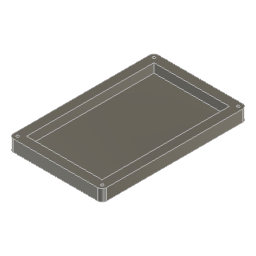
Veekos-bottom (Autodesk Fusion 360 design; units mm, degrees)
part number: 2026-09-15-13-32-07-212
Autodesk Fusion 360 part; units mm, degrees
sketch "Sketch1" plane through (0, 0, 0) normal (0, 0, 1) x (1, 0, 0)
  line L0 (-51.3011, 107.6317) -> (32.8009, 107.6317)
  line L1 (32.8009, 107.6317) -> (32.8009, -34.1263)
  line L2 (32.8009, -34.1263) -> (-51.3011, -34.1263)
  line L3 (-51.3011, -34.1263) -> (-51.3011, 107.6317)
  line L4 (-61.3011, 117.6317) -> (42.8009, 117.6317)
  line L5 (42.8009, 117.6317) -> (42.8009, -44.1263)
  line L6 (42.8009, -44.1263) -> (-61.3011, -44.1263)
  line L7 (-61.3011, -44.1263) -> (-61.3011, 117.6317)
  circle A0 centre (37.8009, 112.6317) radius 1.45
  circle A1 centre (37.8009, -39.1263) radius 1.45
  circle A2 centre (-56.3011, -39.1263) radius 1.45
  circle A3 centre (-56.3011, 112.6317) radius 1.45
  dimension "d1" = 84.102
  dimension "d2" = 141.758
  dimension "d3" = 104.102
  dimension "d4" = 161.758
  dimension "d5" = 10
  dimension "d6" = 10
  dimension "d7" = 2.9
  dimension "d8" = 5
  dimension "d9" = 5
  dimension "d10" = 2.9
  dimension "d11" = 5
  dimension "d12" = 5
  dimension "d13" = 2.9
  dimension "d14" = 5
  dimension "d15" = 5
  dimension "d16" = 2.9
  dimension "d17" = 5
  dimension "d18" = 5
  constraint horizontal L0
  constraint vertical L1
  constraint horizontal L2
  constraint vertical L3
  constraint horizontal L4
  constraint vertical L5
  constraint horizontal L6
  constraint vertical L7
  measures "d1" distance of L0.start L0.end
  measures "d2" distance of L0.start L2.end
  measures "d3" distance of L4.start L4.end
  measures "d4" distance of L4.start L6.end
  measures "d5" distance of L0 L4
  measures "d6" distance of L3 L7
  measures "d7" diameter of A0
  measures "d8" distance of L5 A0.centre
  measures "d9" distance of L4 A0.centre
  measures "d10" diameter of A1
  measures "d11" distance of L6 A1.centre
  measures "d12" distance of L5 A1.centre
  measures "d13" diameter of A2
  measures "d14" distance of L7 A2.centre
  measures "d15" distance of L6 A2.centre
  measures "d16" diameter of A3
  measures "d17" distance of L4 A3.centre
  measures "d18" distance of L7 A3.centre
extrude "Extrude1" add sketch "Sketch1" along normal blind 3 contours L0 L1 L2 L3
extrude "Extrude2" add sketch "Sketch1" along normal blind 13
fillet "Fillet1" radius 5 4 edges at (42.8009, -44.1263, 6.5) (42.8009, 117.6317, 6.5) (-61.3011, 117.6317, 6.5) (-61.3011, -44.1263, 6.5)
